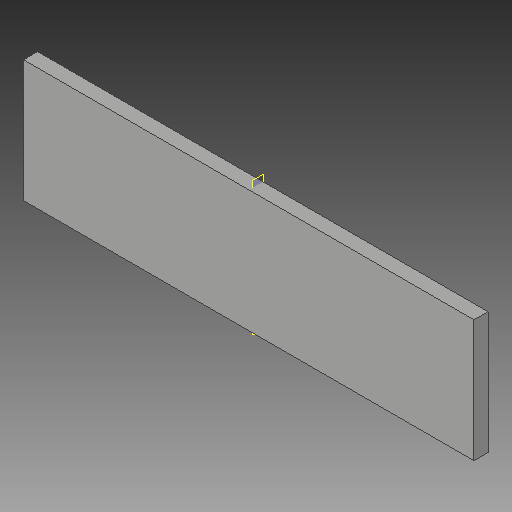
# Autodesk Inventor part: skot opad smal
Saved by Autodesk Inventor 2018 (Build 220112000, 112)
## iProperties
Created: 2019-09-30
Part Number: skot opad smal
Material: S355MC
Document SubType Name: Sheet Metal
Designer: loppen
Density: 7.85 g/cm^3
Sheet Metal Rule: Default_mm
Appearance: Light Gray
Mass: 39.1872 g
Surface Area: 54.8 cm^2
Volume: 4.992 cm^3
Flat Pattern Width: 2.6 cm
Flat Pattern Length: 9.6 cm
Flat Pattern Area: 24.96 cm^2
Sheet Metal Width: 26,000 mm
Sheet Metal Length: 96,000 mm
Sheet Metal Area: 2496,000 mm^2
Author: loppen
Autodesk Inventor part; units mm, degrees
ref_plane "YZ Plane" through (0, 0, 0) normal (1, 0, 0) x (0, 1, 0)
ref_plane "XZ Plane" through (0, 0, 0) normal (0, 1, 0) x (-1, 0, 0)
ref_plane "XY Plane" through (0, 0, 0) normal (0, 0, 1) x (1, 0, 0)
ref_plane "Work Plane1" through (0, 0, 0) normal (0, 0, 1) x (1, 0, 0)
sketch "Sketch1" plane through (0, 0, 0) normal (0, 0, 1) x (1, 0, 0)
  line L0 (-109, -242.4163) -> (-109, -238.4163)
  line L1 (-119, -238.4163) -> (-109, -238.4163)
  arc A0 (-124, -233.4163) -> (-119, -238.4163) centre (-119, -233.4163) ccw
  line L2 (-124, -154.5344) -> (-124, -233.4163)
  arc A1 (-123.8494, -153.3167) -> (-124, -154.5344) centre (-119, -154.5344) ccw
  line L3 (-103.571, -72.5602) -> (-123.8494, -153.3167)
  arc A2 (-103.1284, -71.4158) -> (-103.571, -72.5602) centre (-98.7216, -73.7779) ccw
  line L4 (-68.4069, -6.6379) -> (-103.1284, -71.4158)
  arc A3 (-59.5931, -6.6379) -> (-68.4069, -6.6379) centre (-64, -9) ccw
  line L5 (-24.8716, -71.4158) -> (-59.5931, -6.6379)
  arc A4 (-24.429, -72.5602) -> (-24.8716, -71.4158) centre (-29.2784, -73.7779) ccw
  line L6 (-4.1506, -153.3167) -> (-24.429, -72.5602)
  arc A5 (-4, -154.5344) -> (-4.1506, -153.3167) centre (-9, -154.5344) ccw
  line L7 (-4, -233.4163) -> (-4, -154.5344)
  arc A6 (-9, -238.4163) -> (-4, -233.4163) centre (-9, -233.4163) ccw
  line L8 (-19, -238.4163) -> (-9, -238.4163)
  line L9 (-19, -238.4163) -> (-19, -242.4163)
  line L10 (-9, -242.4163) -> (-19, -242.4163)
  arc A7 (-9, -242.4163) -> (0, -233.4163) centre (-9, -233.4163) ccw
  line L11 (0, -154.5344) -> (0, -233.4163)
  arc A8 (0, -154.5344) -> (-0.271, -152.3425) centre (-9, -154.5344) ccw
  line L12 (-20.5494, -71.586) -> (-0.271, -152.3425)
  arc A9 (-20.5494, -71.586) -> (-21.3461, -69.5261) centre (-29.2784, -73.7779) ccw
  line L13 (-56.0677, -4.7482) -> (-21.3461, -69.5261)
  arc A10 (-56.0677, -4.7482) -> (-71.9323, -4.7482) centre (-64, -9) ccw
  line L14 (-106.6539, -69.5261) -> (-71.9323, -4.7482)
  arc A11 (-106.6539, -69.5261) -> (-107.4506, -71.586) centre (-98.7216, -73.7779) ccw
  line L15 (-127.729, -152.3425) -> (-107.4506, -71.586)
  arc A12 (-127.729, -152.3425) -> (-128, -154.5344) centre (-119, -154.5344) ccw
  line L16 (-128, -233.4163) -> (-128, -154.5344)
  arc A13 (-128, -233.4163) -> (-119, -242.4163) centre (-119, -233.4163) ccw
  line L17 (-109, -242.4163) -> (-119, -242.4163)
  line L18 (-112, -212.4163) -> (-16, -212.4163)
  line L19 (-16, -212.4163) -> (-16, -238.4163)
  line L20 (-16, -238.4163) -> (-112, -238.4163)
  line L21 (-112, -238.4163) -> (-112, -212.4163)
  point P0 (0, 0)
  dimension "d8" = 12
  dimension "d9" = 12
  dimension "d10" = 26
  measures "d8" distance between parallel lines of L2 L21
  measures "d9" distance between parallel lines of L7 L19
  measures "d10" distance between parallel lines of L20 L18
extrude "Plate1" add sketch "Sketch1" along normal blind 3 contours L1 L21 L18 L19 L8 L20
ref_plane "midtplan" through (-64, -238.4163, 0) normal (-1, 0, 0) x (0, 0, 1)
equation "\"d9\" = d8"
equation "\"d7\" = Thickness"
equation "\"Thickness\" = pladetykkelse"
equation "\"BendRadius\" = 1.5 * Thickness"
equation "\"BendReliefWidth\" = Thickness"
equation "\"BendReliefDepth\" = 0.5 * Thickness"
equation "\"CornerReliefSize\" = 4 * Thickness"
equation "\"MinimumRemnant\" = 2 * Thickness"
equation "\"TransitionRadius\" = BendRadius"
equation "\"JacobiRadiusSize\" = BendRadius"
equation "\"GapSize\" = Thickness"
equation "\"pladetykkelse\" = 3"
equation "\"trappevinkel\" = 34.3deg"
equation "\"trappestifter_dia\" = 25"
equation "\"trappestifter_huldia\" = 25.8"
equation "\"trappestifter_skraa_huldia\" = 26.6"
equation "\"trappestifter_laengde\" = 228"
equation "\"perforeringsbredde\" = 6"
equation "\"perforeringshullaengde\" = 62.8"
equation "\"perforeringshullaengde_top\" = 61"
equation "\"perforeringshullaengde_bund\" = 61.6"
equation "\"perforeringsoffset\" = 8"
equation "\"perforeringsoffset_top\" = 8"
equation "\"perforeringsoffset_bund\" = 8"
equation "\"laskehul_dia\" = 13"
equation "\"balusterhul_udvidelse\" = 1"
body "Solid1"
